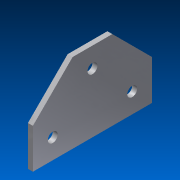
# Autodesk Inventor part: SupportT
Saved by Autodesk Inventor 2013 (Build 170138000, 138)
## iProperties
Created: 2013-07-23
Part Number: SupportT
Material: Aluminum 6061
Document SubType Name: Modeling
Designer: orange
Density: 1 g/cm^3
Author: orange
Autodesk Inventor part; units mm, degrees
ref_plane "YZ Plane" through (0, 0, 0) normal (1, 0, 0) x (0, 1, 0)
ref_plane "XZ Plane" through (0, 0, 0) normal (0, 1, 0) x (-1, 0, 0)
ref_plane "XY Plane" through (0, 0, 0) normal (0, 0, 1) x (1, 0, 0)
sketch "Sketch1" plane through (0, 0, 0) normal (1, 0, 0) x (0, 1, 0)
  line L0 (50.8, 25.4) -> (50.8, 50.8)
  line L1 (50.8, 50.8) -> (25.4, 76.2)
  line L2 (25.4, 76.2) -> (0, 76.2)
  line L3 (0, 76.2) -> (0, 0)
  line L4 (0, 0) -> (25.4, 0)
  line L5 (25.4, 0) -> (50.8, 25.4)
  dimension "d0" = 76.2
  dimension "d1" = 25.4
  dimension "d3" = 25.4
  dimension "d4" = 25.4
  dimension "d5" = 25.4
  dimension "d6" = 25.4
  dimension "d7" = 50.8
  constraints: 12 end point, 1 parallel, 1 perpendicular
  measures "d0" distance of L2.end L3.end
  measures "d1" distance of L0.start L0.end
  measures "d3" distance of L3.end L4.end
  measures "d4" distance of L1.end L2.end
  measures "d5" distance from line of L0.end L2
  measures "d6" distance from line of L4 L0.start
  measures "d7" distance between parallel lines of L3 L0
extrude "Extrusion1" add sketch "Sketch1" along normal blind 3.175
sketch "Sketch2" plane through (3.175, 0, 0) normal (1, 0, 0) x (0, 0, -1)
  line L0 (-76.2, 0) -> (0, 0) projected
  line L1 (0, 0) -> (0, 25.4) projected
  line L2 (-25.4, 50.8) -> (-50.8, 50.8) projected
  line L3 (-76.2, 25.4) -> (-76.2, 0) projected
  point P0 (-38.1, 38.1)
  point P1 (-12.7, 12.7)
  point P2 (-63.5, 12.7)
  dimension "d10" = 12.7
  dimension "d11" = 12.7
  dimension "d12" = 12.7
  dimension "d13" = 12.7
  dimension "d14" = 12.7
  dimension "d15" = 12.7
  measures "d10" distance from line of L0 point (-63.5, 12.7)
  measures "d11" distance from line of L3 point (-63.5, 12.7)
  measures "d12" distance from line of point (-38.1, 38.1) L2
  measures "d13" horizontal distance of L2.end point (-38.1, 38.1)
  measures "d14" distance from line of L1 point (-12.7, 12.7)
  measures "d15" distance from line of point (-12.7, 12.7) L0
hole "Hole1" at (3.175, 38.1, 38.1) at (3.175, 12.7, 12.7) at (3.175, 12.7, 63.5) direction (-1, 0, 0) diameter 6.35 end through all
body "Solid1"
